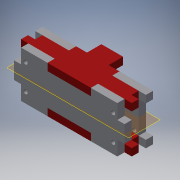
# Autodesk Inventor part: box
Saved by Autodesk Inventor 2019 (Build 230136000, 136)
## iProperties
Created: 2018-09-20
Part Number: box
Material: Générique
Document SubType Name: Modeling
Designer: Jérémy
Density: 1 g/cm^3
Appearance: Par défaut
Author: Jérémy
Autodesk Inventor part; units mm, degrees
ref_plane "YZ Plane" through (0, 0, 0) normal (1, 0, 0) x (0, 1, 0)
ref_plane "XZ Plane" through (0, 0, 0) normal (0, 1, 0) x (-1, 0, 0)
ref_plane "XY Plane" through (0, 0, 0) normal (0, 0, 1) x (1, 0, 0)
sketch "Esquisse1" plane through (0, 0, 0) normal (0, 0, 1) x (1, 0, 0)
  line L0 (0, 11.8) -> (0, 9.4) projected
  line L1 (0, 11.8) -> (-8.8, 11.8) construction
  line L2 (-8.8, 0) -> (-8.8, 11.8) construction
  line L3 (0, 0) -> (-8.8, 0) projected
  line L4 (0, 2.4) -> (0, 0) projected
  line L5 (0, 2.4) -> (19.5, 2.4) projected
  line L6 (19.5, 9.4) -> (19.5, 2.4) projected
  line L7 (0, 9.4) -> (19.5, 9.4) projected
  line L8 (59, 0) -> (59, 2.4) projected
  line L9 (59, 0) -> (67.8, 0) projected
  line L10 (67.8, 11.8) -> (67.8, 0) construction
  line L11 (59, 11.8) -> (67.8, 11.8) construction
  line L12 (59, 9.4) -> (59, 11.8) projected
  line L13 (59, 9.4) -> (39.5, 9.4) projected
  line L14 (39.5, 2.4) -> (39.5, 9.4) projected
  line L15 (59, 2.4) -> (39.5, 2.4) projected
  line L16 (19.5, 9.4) -> (19.5, 5.9) construction
  line L17 (19.5, 5.9) -> (19.5, 2.4) construction
  line L18 (19.5, 9.4) -> (29.5, 9.4) construction
  line L19 (29.5, 9.4) -> (39.5, 9.4) construction
  line L20 (-27.9434, 5.9) -> (85.3545, 5.9) construction
  line L21 (29.5, 17.9523) -> (29.5, -8.6548) construction
  line L22 (-8.8, 5.9) -> (-8.8, 11.8)
  line L23 (-3.8, 11.8) -> (-3.8, 21.9)
  line L24 (-3.8, 21.9) -> (14.5, 21.9)
  line L25 (14.5, 21.9) -> (14.5, 16.9)
  line L26 (14.5, 16.9) -> (29.5, 16.9)
  line L27 (-3.8, 11.8) -> (-8.8, 11.8)
  circle A0 centre (-0.8, 14.8) radius 1.5
  line L28 (59, 11.8) -> (67.8, 11.8) construction
  line L29 (67.8, 0) -> (67.8, 11.8) construction
  line L30 (67.8, 5.9) -> (67.8, 11.8)
  line L31 (62.8, 11.8) -> (62.8, 21.9)
  line L32 (62.8, 21.9) -> (44.5, 21.9)
  line L33 (44.5, 21.9) -> (44.5, 16.9)
  line L34 (44.5, 16.9) -> (29.5, 16.9)
  line L35 (62.8, 11.8) -> (67.8, 11.8)
  circle A1 centre (59.8, 14.8) radius 1.5
  line L36 (0, 0) -> (-8.8, 0) construction
  line L37 (59, 0) -> (67.8, 0) construction
  line L38 (-8.8, 5.9) -> (-8.8, 0)
  line L39 (-3.8, 0) -> (-3.8, -10.1)
  line L40 (-3.8, -10.1) -> (14.5, -10.1)
  line L41 (14.5, -10.1) -> (14.5, -5.1)
  line L42 (14.5, -5.1) -> (29.5, -5.1)
  line L43 (-3.8, 0) -> (-8.8, 0)
  circle A2 centre (-0.8, -3) radius 1.5
  line L44 (59, 0) -> (67.8, 0) construction
  line L45 (62.8, -10.1) -> (44.5, -10.1)
  line L46 (44.5, -5.1) -> (29.5, -5.1)
  line L47 (44.5, -10.1) -> (44.5, -5.1)
  circle A3 centre (59.8, -3) radius 1.5
  line L48 (62.8, 0) -> (62.8, -10.1)
  line L49 (62.8, 0) -> (67.8, 0)
  line L50 (67.8, 5.9) -> (67.8, 0)
  point P0 (19.5, 5.9)
  dimension "d0" = 5
  dimension "d1" = 15
  dimension "d2" = 5
  dimension "d3" = 16
  dimension "d4" = 3
  dimension "d5" = 3
  dimension "d6" = 3
  constraints: 70 end point, 17 symmetric about line, 8 point on line, 6 collinear, 4 centre point, 4 perpendicular, 3 midpoint, 2 coincident, 1 horizontal, 1 parallel, 1 vertical, 3 other
  measures "d0" distance of L1.end L23.start
  measures "d1" distance of L25.end L26.end
  measures "d2" distance of L24.end L25.end
  measures "d3" vertical distance of L22.start L23.end
  measures "d4" diameter of A0
  measures "d5" vertical distance of L0.start A0.centre
  measures "d6" horizontal distance of L23.start A0.centre
extrude "Extrusion1" add sketch "Esquisse1" along normal blind 5
ref_plane "Plan de construction1" through (0, 11.8, -9.8) normal (0, 0, -1) x (-1, 0, 0)
sketch "Esquisse2" plane through (0, 11.8, -9.8) normal (0, 0, -1) x (-1, 0, 0)
  circle A0 centre (-59.8, -14.8) radius 1.5 projected
  circle A1 centre (0.8, -14.8) radius 1.5 projected
  circle A2 centre (-59.8, 3) radius 1.5 projected
  circle A3 centre (0.8, 3) radius 1.5 projected
  line L0 (8.8, 0) -> (8.8, -11.8) projected
  line L1 (3.8, 0) -> (8.8, 0) projected
  line L2 (3.8, 10.1) -> (3.8, 0) projected
  line L3 (-14.5, 10.1) -> (3.8, 10.1) projected
  line L4 (-14.5, 5.1) -> (-14.5, 10.1) projected
  line L5 (-44.5, 5.1) -> (-14.5, 5.1) projected
  line L6 (-44.5, 10.1) -> (-44.5, 5.1) projected
  line L7 (-62.8, 10.1) -> (-44.5, 10.1) projected
  line L8 (-62.8, 0) -> (-62.8, 10.1) projected
  line L9 (-67.8, 0) -> (-62.8, 0) projected
  line L10 (-67.8, -11.8) -> (-67.8, 0) projected
  line L11 (-62.8, -11.8) -> (-67.8, -11.8) projected
  line L12 (-62.8, -21.9) -> (-62.8, -11.8) projected
  line L13 (-44.5, -21.9) -> (-62.8, -21.9) projected
  line L14 (-44.5, -16.9) -> (-44.5, -21.9) projected
  line L15 (-14.5, -16.9) -> (-44.5, -16.9) construction
  line L16 (-14.5, -21.9) -> (-14.5, -16.9) projected
  line L17 (3.8, -21.9) -> (-14.5, -21.9) projected
  line L18 (3.8, -11.8) -> (3.8, -21.9) construction
  line L19 (8.8, -11.8) -> (3.8, -11.8) projected
  line L20 (-67.8, -11.8) -> (-67.8, 0) construction
  line L21 (-67.8, -11.8) -> (-67.8, -5.9) construction
  line L22 (-67.8, -5.9) -> (-67.8, 0) construction
  line L23 (23.1291, -5.9) -> (-93.9049, -5.9) construction
  line L24 (-14.5, -16.9) -> (-44.5, -16.9) construction
  line L25 (-14.5, -16.9) -> (-29.5, -16.9) construction
  line L26 (-29.5, -16.9) -> (-44.5, -16.9) construction
  line L27 (-29.5, -48.0449) -> (-29.5, 22.4449) construction
  line L28 (8.8, -21.9) -> (8.8, -16.85)
  line L29 (8.8, -16.85) -> (3.8, -16.85)
  line L30 (3.8, -5.9) -> (3.8, -16.85)
  line L31 (3.8, -21.9) -> (-14.5, -21.9) projected
  line L32 (8.8, -21.9) -> (-14.5, -21.9)
  line L33 (-14.5, -21.9) -> (-14.5, -16.9)
  line L34 (-29.5, -16.9) -> (-14.5, -16.9)
  line L35 (-14.5, -16.9) -> (18.1212, -16.9) construction
  line L36 (-14.5, -11.8) -> (-14.5, 0) construction
  line L37 (-14.5, 0) -> (-19.5, 0) construction
  line L38 (-19.5, -11.8) -> (-19.5, 0) construction
  line L39 (-14.5, -11.8) -> (-19.5, -11.8) construction
  line L40 (-44.5, 0) -> (-44.5, -11.8) construction
  line L41 (-44.5, -11.8) -> (-39.5, -11.8) construction
  line L42 (-39.5, 0) -> (-39.5, -11.8) construction
  line L43 (-44.5, 0) -> (-39.5, 0) construction
  line L44 (-29.5, -12.8) -> (-12.5, -12.8)
  line L45 (-12.5, -12.8) -> (-12.5, -12.8)
  line L46 (-12.5, -12.8) -> (-12.5, -5.9)
  circle A4 centre (-59.8, -14.8) radius 1.5
  line L47 (-44.5, -16.9) -> (-14.5, -16.9) construction
  line L48 (-44.5, -21.9) -> (-44.5, -16.9)
  line L49 (-62.8, -21.9) -> (-44.5, -21.9)
  line L50 (-44.5, -16.9) -> (-14.5, -16.9) construction
  line L51 (-44.5, -16.9) -> (-29.5, -16.9) construction
  line L52 (-67.8, -21.9) -> (-67.8, -16.85)
  line L53 (-67.8, -16.85) -> (-62.8, -16.85)
  line L54 (-62.8, -5.9) -> (-62.8, -16.85)
  line L55 (-67.8, -21.9) -> (-44.5, -21.9)
  line L56 (-29.5, -16.9) -> (-44.5, -16.9)
  line L57 (-29.5, -12.8) -> (-46.5, -12.8)
  line L58 (-46.5, -12.8) -> (-46.5, -5.9)
  circle A5 centre (-59.8, 3) radius 1.5
  circle A6 centre (0.8, 3) radius 1.5
  line L59 (-44.5, 10.1) -> (-62.8, 10.1)
  line L60 (-44.5, 5.1) -> (-44.5, 10.1)
  line L61 (-14.5, 10.1) -> (-14.5, 5.1)
  line L62 (3.8, 10.1) -> (-14.5, 10.1)
  line L63 (3.8, 0) -> (3.8, 10.1) construction
  line L64 (-14.5, 5.1) -> (-29.5, 5.1) construction
  line L65 (8.8, 10.1) -> (8.8, 5.05)
  line L66 (8.8, 5.05) -> (3.8, 5.05)
  line L67 (3.8, -5.9) -> (3.8, 5.05)
  line L68 (3.8, 10.1) -> (-14.5, 10.1)
  line L69 (8.8, 10.1) -> (-14.5, 10.1)
  line L70 (-14.5, 10.1) -> (-14.5, 5.1)
  line L71 (-29.5, 5.1) -> (-14.5, 5.1)
  line L72 (-29.5, 1) -> (-12.5, 1)
  line L73 (-12.5, 1) -> (-12.5, -5.9)
  line L74 (-29.5, 5.1) -> (-44.5, 5.1)
  line L75 (-67.8, 10.1) -> (-44.5, 10.1)
  line L76 (-67.8, 10.1) -> (-67.8, 5.05)
  line L77 (-67.8, 5.05) -> (-62.8, 5.05)
  line L78 (-62.8, -5.9) -> (-62.8, 5.05)
  line L79 (-46.5, 1) -> (-46.5, -5.9)
  line L80 (-29.5, 1) -> (-46.5, 1)
  circle A7 centre (-59.8, 3) radius 1.5
  point P0 (0, -11.8)
  dimension "d9" = 2
  dimension "d10" = 1
  constraints: 100 end point, 26 symmetric about line, 7 point on line, 6 collinear, 4 centre point, 4 midpoint, 4 perpendicular, 2 coincident, 2 parallel, 1 horizontal, 1 vertical, 4 other
  measures "d9" distance between parallel lines of L46 L36
  measures "d10" distance between parallel lines of L39 L44
extrude "Extrusion2" add sketch "Esquisse2" along normal blind 5 contours L67 L30 L29 L28 L32 L17 L16 L34 L56 L14 L13 L12 L54 L78 L8 L7 L6 L5 L4 L3 L2 | L2 L69 L65 L66 | L8 L77 L76 L75 | L55 L52 L53 L12
ref_plane "Plan de construction2" through (-8.8, 5.9, -9.8) normal (0, 1, 0) x (1, 0, 0)
sketch "Esquisse6" plane through (-8.8, 21.9, -9.8) normal (0, 1, 0) x (1, 0, 0)
  line L0 (23.3, 0) -> (53.3, 0) construction
  line L1 (53.3, 0) -> (53.3, 5) construction
  line L2 (23.3, 5) -> (53.3, 5) construction
  line L3 (23.3, 0) -> (23.3, 5) construction
  line L4 (0, 0) -> (23.3, 0) construction
  line L5 (23.3, 0) -> (23.3, 5) construction
  line L6 (0, 5) -> (23.3, 5) construction
  line L7 (0, 0) -> (0, 5) construction
  line L8 (53.3, 0) -> (76.6, 0) construction
  line L9 (76.6, 0) -> (76.6, 5) construction
  line L10 (53.3, 5) -> (76.6, 5) construction
  line L11 (53.3, 0) -> (53.3, 5) construction
  line L12 (71.6, -9.8) -> (53.3, -9.8) construction
  line L13 (53.3, -9.8) -> (53.3, -14.8) construction
  line L14 (71.6, -14.8) -> (53.3, -14.8) construction
  line L15 (71.6, -9.8) -> (71.6, -14.8) construction
  line L16 (53.3, -9.8) -> (23.3, -9.8) construction
  line L17 (23.3, -9.8) -> (23.3, -14.8) construction
  line L18 (53.3, -14.8) -> (23.3, -14.8) construction
  line L19 (53.3, -9.8) -> (53.3, -14.8) construction
  line L20 (23.3, -9.8) -> (5, -9.8) construction
  line L21 (5, -9.8) -> (5, -14.8) construction
  line L22 (23.3, -14.8) -> (5, -14.8) construction
  line L23 (23.3, -9.8) -> (23.3, -14.8) construction
  line L24 (23.3, -9.8) -> (5, -9.8) projected
  line L25 (5, -9.8) -> (0, -9.8)
  line L26 (0, 0) -> (0, -14.8) construction
  line L27 (0, 0) -> (23.3, 0) construction
  line L28 (5, -9.8) -> (0, -9.8) projected
  line L29 (0, -9.8) -> (0, -5)
  line L30 (0, -5) -> (5, -5)
  line L31 (5, -5) -> (5, 0)
  line L32 (5, 0) -> (23.3, 0)
  line L33 (23.3, 0) -> (23.3, 5) projected
  line L34 (23.3, 0) -> (23.3, 5)
  line L35 (53.3, 0) -> (53.3, 5) projected
  line L36 (53.3, 5) -> (53.3, 0)
  line L37 (5, -9.8) -> (23.3, -9.8)
  line L38 (23.3, -9.8) -> (23.3, -14.8)
  line L39 (23.3, -14.8) -> (5, -14.8) projected
  line L40 (53.3, -14.8) -> (53.3, -9.8)
  line L41 (53.3, -9.8) -> (53.3, -14.8) projected
  line L42 (53.3, -9.8) -> (76.6, -9.8)
  line L43 (76.6, -9.8) -> (76.6, -5)
  line L44 (76.6, -5) -> (71.6, -5)
  line L45 (71.6, -5) -> (71.6, 0)
  line L46 (53.3, 0) -> (76.6, 0) projected
  line L47 (53.3, 0) -> (71.6, 0)
  line L48 (76.6, 0) -> (76.6, 5) projected
  line L49 (23.3, 0) -> (23.3, 5) projected
  line L50 (23.3, 5) -> (38.3, 5) construction
  line L51 (38.3, 5) -> (53.3, 5) construction
  line L52 (38.3, 17.4784) -> (38.3, -29.8094) construction
  line L53 (45.8, 15) -> (45.8, 5)
  line L54 (53.3, 5) -> (45.8, 5)
  line L55 (30.8, 15) -> (38.3, 15)
  line L56 (38.3, 15) -> (45.8, 15)
  line L57 (23.3, 5) -> (53.3, 5) projected
  line L58 (23.3, 5) -> (30.8, 5)
  line L59 (30.8, 15) -> (30.8, 5)
  line L60 (53.3, -14.8) -> (71.6, -14.8) projected
  line L61 (23.3, -14.8) -> (53.3, -14.8)
  point P0 (8.8, -9.8)
  dimension "d28" = 5
  dimension "d29" = 5
  dimension "d33" = 10
  dimension "d35" = 7.5
  constraints: 52 end point, 7 collinear, 7 perpendicular, 6 horizontal, 6 point on line, 4 parallel, 2 midpoint, 1 coincident, 1 vertical, 2 other
  measures "d28" distance of L44.end L45.end
  measures "d29" distance of L43.end L44.end
  measures "d33" distance of L53.start L53.end
  measures "d35" distance of L55.end L53.start
extrude "Extrusion4" add sketch "Esquisse6" against normal blind 5 separate body
mirror "Symétrie2" about plane through (-8.8, 5.9, -9.8) normal (0, 1, 0) of "Extrusion4" bodies 2
equation "\"d0\" = epaisseur"
equation "\"d1\" = 0.5 * L_fente"
equation "\"d2\" = epaisseur"
equation "\"d3\" = 0.5 * largeur"
equation "\"d4\" = dvis"
equation "\"d5\" = dvis"
equation "\"d6\" = dvis"
equation "\"d7\" = epaisseur"
equation "\"d11\" = epaisseur"
equation "\"d28\" = epaisseur"
equation "\"d29\" = epaisseur"
equation "\"d33\" = epaisseur + marge_attache_carte"
equation "\"d35\" = 0.5 * L_attache_carte"
equation "\"d30\" = epaisseur"
equation "\"epaisseur\" = 5"
equation "\"dvis\" = 3"
equation "\"largeur\" = 32"
equation "\"L_attache_carte\" = 15"
equation "\"marge_attache_carte\" = 5"
equation "\"taille_trou\" = 7"
equation "\"L_moteur\" = 28.3"
equation "\"largeur_cubi\" = 76.6"
equation "\"marge_trou\" = 2"
equation "\"L_cubi\" = 76.6"
equation "\"L_fente\" = 30"
